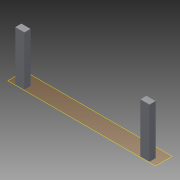
# Autodesk Inventor part: CrossBeam2
Saved by Autodesk Inventor 2014 SP1 (Build 180222100, 222)
## iProperties
Created: 2017-05-21
Part Number: CrossBeam2
Material: Generic
Document SubType Name: Modeling
Designer: danielsikar
Density: 1 g/cm^3
Appearance: Default
Author: danielsikar
Autodesk Inventor part; units mm, degrees
ref_plane "YZ Plane" through (0, 0, 0) normal (1, 0, 0) x (0, 1, 0)
ref_plane "XZ Plane" through (0, 0, 0) normal (0, 1, 0) x (-1, 0, 0)
ref_plane "Work Plane1" through (0, 0, 0) normal (0, 0, 1) x (1, 0, 0)
sketch "Sketch1" plane through (0, 0, 0) normal (0, 0, 1) x (1, 0, 0)
  line L0 (-9.5, 4) -> (-78.7, 4) construction
  line L1 (0, 0) -> (-88.2, 0) construction
  line L2 (-88.2, 0) -> (-88.2, 10) construction
  line L3 (-88.2, 4) -> (-82.2, 4)
  line L4 (-82.2, 4) -> (-82.2, 0)
  line L5 (-82.2, 0) -> (-88.2, 0)
  line L6 (-88.2, 0) -> (-88.2, 4)
  line L7 (-6, 4) -> (0, 4)
  line L8 (0, 4) -> (0, 0)
  line L9 (0, 0) -> (-6, 0)
  line L10 (-6, 0) -> (-6, 4)
  line L11 (0, 0) -> (0, 10) construction
  dimension "d0" = 6
  dimension "d1" = 6
  dimension "d2" = 0
  dimension "d3" = 0
  constraints: 16 end point, 4 parallel, 4 point on line, 2 horizontal, 2 perpendicular
  measures "d0" distance of L4.end L5.end
  measures "d1" distance of L8.end L9.end
  measures "d2" distance between parallel lines of L11 L8
  measures "d3" distance between parallel lines of L6 L2
ref_plane "Work Plane2" through (-88.2, 0, 32.5) normal (0, 0, -1) x (0, 1, 0)
extrude "Extrusion1" add sketch "Sketch1" along normal up to surface (32.5 mm away)
body "Solid1"
